Autodesk Fusion 360 part; units mm, degrees
note: some values were not read from the file. Set by a fixed rule: which sketch regions a step uses.
(part 2 of 2)
sketch "Sketch8" plane through (0, 0, 0) normal (1, 0, 0) x (0, 1, 0)
  spline S0 degree 3 poles (29.3326, 12.3675) (29.5623, 12.3811) (30.0065, 12.4074) (30.3868, 12.6373) (30.5704, 12.7484) knots 0 0 0 0 0.067871 0.131252 0.131252 0.131252 0.131252
  spline S1 degree 3 poles (30.5704, 12.7484) (30.736, 12.9046) (31.0986, 13.2469) (31.2831, 13.7117) (31.3834, 13.9642) knots 0 0 0 0 0.067501 0.147835 0.147835 0.147835 0.147835
  line L0 (31.3834, 13.9642) -> (32.7457, 13.7957)
  spline S2 degree 3 poles (32.7457, 13.7957) (32.6206, 13.424) (32.3783, 12.7048) (31.8211, 12.191) (31.5519, 11.9427) knots 0 0 0 0 0.115551 0.223613 0.223613 0.223613 0.223613
  spline S3 degree 3 poles (31.5519, 11.9427) (31.2294, 11.7506) (30.5449, 11.3428) (29.7472, 11.304) (29.3253, 11.2835) knots 0 0 0 0 0.110875 0.235384 0.235384 0.235384 0.235384
  spline S4 degree 3 poles (29.3253, 11.2835) (28.7944, 11.3187) (27.7792, 11.386) (26.9937, 12.0282) (26.619, 12.3345) knots 0 0 0 0 0.155225 0.296837 0.296837 0.296837 0.296837
  spline S5 degree 3 poles (26.619, 12.3345) (26.3278, 12.7407) (25.6988, 13.6182) (25.647, 14.701) (25.6192, 15.2825) knots 0 0 0 0 0.146839 0.31723 0.31723 0.31723 0.31723
  spline S6 degree 3 poles (25.6192, 15.2825) (25.6467, 15.8834) (25.6976, 16.9987) (26.3357, 17.9094) (26.63, 18.3294) knots 0 0 0 0 0.176138 0.326947 0.326947 0.326947 0.326947
  spline S7 degree 3 poles (26.63, 18.3294) (26.998, 18.6455) (27.752, 19.2931) (28.7442, 19.3727) (29.2521, 19.4134) knots 0 0 0 0 0.141726 0.290335 0.290335 0.290335 0.290335
  spline S8 degree 3 poles (29.2521, 19.4134) (29.7447, 19.3729) (30.7102, 19.2935) (31.4423, 18.6611) (31.8009, 18.3514) knots 0 0 0 0 0.144189 0.28257 0.28257 0.28257 0.28257
  spline S9 degree 3 poles (31.8009, 18.3514) (32.0888, 17.9395) (32.7134, 17.046) (32.763, 15.9525) (32.7897, 15.3631) knots 0 0 0 0 0.147764 0.320562 0.320562 0.320562 0.320562
  spline S10 degree 3 poles (32.7897, 15.3631) (32.7892, 15.3143) (32.7881, 15.1971) (32.7845, 15.0799) (32.7823, 15.0115) knots 0 0 0 0 0.01465 0.035165 0.035165 0.035165 0.035165
  line L1 (32.7823, 15.0115) -> (26.9816, 15.0115)
  spline S11 degree 3 poles (26.9816, 15.0115) (27.0197, 14.621) (27.0899, 13.9004) (27.5129, 13.3162) (27.7067, 13.0487) knots 0 0 0 0 0.115238 0.212619 0.212619 0.212619 0.212619
  spline S12 degree 3 poles (27.7067, 13.0487) (27.9388, 12.85) (28.4075, 12.449) (29.0224, 12.3948) (29.3326, 12.3675) knots 0 0 0 0 0.089299 0.180262 0.180262 0.180262 0.180262
  line L2 (61.3028, 12.9608) -> (61.3028, 11.4593)
  line L3 (61.3028, 11.4593) -> (59.7867, 11.4593)
  line L4 (59.7867, 11.4593) -> (59.7867, 12.9608)
  line L5 (59.7867, 12.9608) -> (61.3028, 12.9608)
  spline S13 degree 3 poles (54.2203, 11.2762) (53.7345, 11.3177) (52.7869, 11.3986) (52.1108, 12.0648) (51.7814, 12.3895) knots 0 0 0 0 0.141377 0.275753 0.275753 0.275753 0.275753
  spline S14 degree 3 poles (51.7814, 12.3895) (51.4733, 12.9652) (50.7483, 14.3203) (50.7299, 15.8658) (50.7193, 16.7547) knots 0 0 0 0 0.193319 0.455045 0.455045 0.455045 0.455045
  spline S15 degree 3 poles (50.7193, 16.7547) (50.7271, 17.3309) (50.7411, 18.3686) (50.9973, 19.3732) (51.1112, 19.8199) knots 0 0 0 0 0.172123 0.309967 0.309967 0.309967 0.309967
  spline S16 degree 3 poles (51.1112, 19.8199) (51.25, 20.1782) (51.5131, 20.8578) (52.0309, 21.369) (52.2757, 21.6107) knots 0 0 0 0 0.113767 0.215777 0.215777 0.215777 0.215777
  spline S17 degree 3 poles (52.2757, 21.6107) (52.5579, 21.7943) (53.1481, 22.1784) (53.8526, 22.2192) (54.2203, 22.2405) knots 0 0 0 0 0.099218 0.207577 0.207577 0.207577 0.207577
  spline S18 degree 3 poles (54.2203, 22.2405) (54.4947, 22.2286) (55.0219, 22.2056) (55.5048, 21.9941) (55.7364, 21.8926) knots 0 0 0 0 0.081581 0.15675 0.15675 0.15675 0.15675
  spline S19 degree 3 poles (55.7364, 21.8926) (55.9453, 21.7623) (56.3691, 21.4978) (56.6637, 21.094) (56.8131, 20.8892) knots 0 0 0 0 0.073116 0.148395 0.148395 0.148395 0.148395
  spline S20 degree 3 poles (56.8131, 20.8892) (56.949, 20.651) (57.2368, 20.1465) (57.3957, 19.5875) (57.4796, 19.2926) knots 0 0 0 0 0.081981 0.173584 0.173584 0.173584 0.173584
  spline S21 degree 3 poles (57.4796, 19.2926) (57.5498, 18.9252) (57.71, 18.0874) (57.7172, 17.234) (57.7213, 16.7547) knots 0 0 0 0 0.111981 0.255389 0.255389 0.255389 0.255389
  spline S22 degree 3 poles (57.7213, 16.7547) (57.7135, 16.1822) (57.6993, 15.1497) (57.446, 14.1497) (57.3331, 13.7042) knots 0 0 0 0 0.171021 0.308449 0.308449 0.308449 0.308449
  spline S23 degree 3 poles (57.3331, 13.7042) (57.1953, 13.3456) (56.9337, 12.665) (56.4168, 12.1523) (56.1722, 11.9097) knots 0 0 0 0 0.113733 0.215887 0.215887 0.215887 0.215887
  spline S24 degree 3 poles (56.1722, 11.9097) (55.8896, 11.7251) (55.2975, 11.3382) (54.59, 11.2975) (54.2203, 11.2762) knots 0 0 0 0 0.09951 0.208425 0.208425 0.208425 0.208425
  line L6 (61.3614, 19.8162) -> (60.9806, 14.1253)
  line L7 (60.9806, 14.1253) -> (60.131, 14.1253)
  line L8 (60.131, 14.1253) -> (59.7281, 19.8162)
  line L9 (59.7281, 19.8162) -> (59.7281, 22.1966)
  line L10 (59.7281, 22.1966) -> (61.3614, 22.1966)
  line L11 (61.3614, 22.1966) -> (61.3614, 19.8162)
  line L12 (49.5621, 12.7264) -> (49.5621, 11.4593)
  line L13 (49.5621, 11.4593) -> (42.8531, 11.4593)
  line L14 (42.8531, 11.4593) -> (42.8531, 22.1966)
  line L15 (42.8531, 22.1966) -> (44.274, 22.1966)
  line L16 (44.274, 22.1966) -> (44.274, 12.7264)
  line L17 (44.274, 12.7264) -> (49.5621, 12.7264)
  line L18 (41.2198, 12.7264) -> (41.2198, 11.4593)
  line L19 (41.2198, 11.4593) -> (34.5109, 11.4593)
  line L20 (34.5109, 11.4593) -> (34.5109, 22.1966)
  line L21 (34.5109, 22.1966) -> (35.9317, 22.1966)
  line L22 (35.9317, 22.1966) -> (35.9317, 12.7264)
  line L23 (35.9317, 12.7264) -> (41.2198, 12.7264)
  line L24 (16.8595, 16.5203) -> (16.8595, 11.4593)
  line L25 (16.8595, 11.4593) -> (15.4386, 11.4593)
  line L26 (15.4386, 11.4593) -> (15.4386, 22.1966)
  line L27 (15.4386, 22.1966) -> (16.8595, 22.1966)
  line L28 (16.8595, 22.1966) -> (16.8595, 17.7874)
  line L29 (16.8595, 17.7874) -> (22.4405, 17.7874)
  line L30 (22.4405, 17.7874) -> (22.4405, 22.1966)
  line L31 (22.4405, 22.1966) -> (23.8614, 22.1966)
  line L32 (23.8614, 22.1966) -> (23.8614, 11.4593)
  line L33 (23.8614, 11.4593) -> (22.4405, 11.4593)
  line L34 (22.4405, 11.4593) -> (22.4405, 16.5203)
  line L35 (22.4405, 16.5203) -> (16.8595, 16.5203)
  line L36 (24.5, 46.5) -> (51.5, 46.5)
  line L37 (51.5, 46.5) -> (51.5, 43.5)
  arc A0 (44.0625, 39.115) -> (51.5, 43.5) centre (51.5, 35) ccw
  line L38 (44.0625, 39.115) -> (31.9375, 39.115)
  arc A1 (24.5, 43.5) -> (31.9375, 39.115) centre (24.5, 35) ccw
  line L39 (24.5, 43.5) -> (24.5, 46.5)
  line L40 (63, 56) -> (53, 56)
  line L41 (53, 56) -> (53, 53)
  line L42 (53, 53) -> (43, 53)
  line L43 (43, 53) -> (43, 56)
  line L44 (43, 56) -> (33, 56)
  line L45 (33, 56) -> (33, 53)
  line L46 (33, 53) -> (23, 53)
  line L47 (23, 53) -> (23, 56)
  line L48 (23, 56) -> (13, 56)
  line L49 (13, 56) -> (13, 53)
  line L50 (13, 53) -> (3, 53)
  line L51 (3, 53) -> (3, 56)
  line L52 (3, 56) -> (0, 56)
  line L53 (0, 56) -> (0, 43)
  line L54 (0, 43) -> (3, 43)
  line L55 (3, 43) -> (3, 33)
  line L56 (3, 33) -> (0, 33)
  line L57 (0, 33) -> (0, 23)
  line L58 (0, 23) -> (3, 23)
  line L59 (3, 23) -> (3, 13)
  line L60 (3, 13) -> (0, 13)
  line L61 (0, 13) -> (0, 0)
  line L62 (0, 0) -> (3, 0)
  line L63 (3, 0) -> (3, 3)
  line L64 (3, 3) -> (13, 3)
  line L65 (13, 3) -> (13, 0)
  line L66 (13, 0) -> (23, 0)
  line L67 (23, 0) -> (23, 3)
  line L68 (23, 3) -> (33, 3)
  line L69 (33, 3) -> (33, 0)
  line L70 (33, 0) -> (43, 0)
  line L71 (43, 0) -> (43, 3)
  line L72 (43, 3) -> (53, 3)
  line L73 (53, 3) -> (53, 0)
  line L74 (53, 0) -> (63, 0)
  line L75 (63, 0) -> (63, 3)
  line L76 (63, 3) -> (73, 3)
  line L77 (73, 3) -> (73, 0)
  line L78 (73, 0) -> (76, 0)
  line L79 (76, 0) -> (76, 13)
  line L80 (76, 13) -> (73, 13)
  line L81 (73, 13) -> (73, 23)
  line L82 (73, 23) -> (76, 23)
  line L83 (76, 23) -> (76, 33)
  line L84 (76, 33) -> (73, 33)
  line L85 (73, 33) -> (73, 43)
  line L86 (73, 43) -> (76, 43)
  line L87 (76, 43) -> (76, 56)
  line L88 (76, 56) -> (73, 56)
  line L89 (73, 56) -> (73, 53)
  line L90 (73, 53) -> (63, 53)
  line L91 (63, 53) -> (63, 56)
sketch "Sketch9" plane through (0, 76, 0) normal (0, 1, 0) x (-1, 0, 0)
  line L0 (183, 0) -> (193, 0)
  line L1 (193, 0) -> (193, 13)
  line L2 (193, 13) -> (196, 13)
  line L3 (196, 13) -> (196, 23)
  line L4 (196, 23) -> (193, 23)
  line L5 (193, 23) -> (193, 33)
  line L6 (193, 33) -> (196, 33)
  line L7 (196, 33) -> (196, 43)
  line L8 (196, 43) -> (193, 43)
  line L9 (193, 43) -> (193, 56)
  line L10 (193, 56) -> (183, 56)
  line L11 (183, 56) -> (183, 53)
  line L12 (183, 53) -> (173, 53)
  line L13 (173, 53) -> (173, 56)
  line L14 (173, 56) -> (163, 56)
  line L15 (163, 56) -> (163, 53)
  line L16 (163, 53) -> (153, 53)
  line L17 (153, 53) -> (153, 56)
  line L18 (153, 56) -> (143, 56)
  line L19 (143, 56) -> (143, 53)
  line L20 (143, 53) -> (133, 53)
  line L21 (133, 53) -> (133, 56)
  line L22 (133, 56) -> (123, 56)
  line L23 (123, 56) -> (123, 53)
  line L24 (123, 53) -> (113, 53)
  line L25 (113, 53) -> (113, 56)
  line L26 (113, 56) -> (103, 56)
  line L27 (103, 56) -> (103, 53)
  line L28 (103, 53) -> (93, 53)
  line L29 (93, 53) -> (93, 56)
  line L30 (93, 56) -> (83, 56)
  line L31 (83, 56) -> (83, 53)
  line L32 (83, 53) -> (73, 53)
  line L33 (73, 53) -> (73, 56)
  line L34 (73, 56) -> (63, 56)
  line L35 (63, 56) -> (63, 53)
  line L36 (63, 53) -> (53, 53)
  line L37 (53, 53) -> (53, 56)
  line L38 (53, 56) -> (43, 56)
  line L39 (43, 56) -> (43, 53)
  line L40 (43, 53) -> (33, 53)
  line L41 (33, 53) -> (33, 56)
  line L42 (33, 56) -> (23, 56)
  line L43 (23, 56) -> (23, 53)
  line L44 (23, 53) -> (13, 53)
  line L45 (13, 53) -> (13, 56)
  line L46 (13, 56) -> (3, 56)
  line L47 (3, 56) -> (3, 43)
  line L48 (3, 43) -> (0, 43)
  line L49 (0, 43) -> (0, 33)
  line L50 (0, 33) -> (3, 33)
  line L51 (3, 33) -> (3, 23)
  line L52 (3, 23) -> (0, 23)
  line L53 (0, 23) -> (0, 13)
  line L54 (0, 13) -> (3, 13)
  line L55 (3, 13) -> (3, 0)
  line L56 (3, 0) -> (13, 0)
  line L57 (13, 0) -> (13, 3)
  line L58 (13, 3) -> (23, 3)
  line L59 (23, 3) -> (23, 0)
  line L60 (23, 0) -> (33, 0)
  line L61 (33, 0) -> (33, 3)
  line L62 (33, 3) -> (43, 3)
  line L63 (43, 3) -> (43, 0)
  line L64 (43, 0) -> (53, 0)
  line L65 (53, 0) -> (53, 3)
  line L66 (53, 3) -> (63, 3)
  line L67 (63, 3) -> (63, 0)
  line L68 (63, 0) -> (73, 0)
  line L69 (73, 0) -> (73, 3)
  line L70 (73, 3) -> (83, 3)
  line L71 (83, 3) -> (83, 0)
  line L72 (83, 0) -> (93, 0)
  line L73 (93, 0) -> (93, 3)
  line L74 (93, 3) -> (103, 3)
  line L75 (103, 3) -> (103, 0)
  line L76 (103, 0) -> (113, 0)
  line L77 (113, 0) -> (113, 3)
  line L78 (113, 3) -> (123, 3)
  line L79 (123, 3) -> (123, 0)
  line L80 (123, 0) -> (133, 0)
  line L81 (133, 0) -> (133, 3)
  line L82 (133, 3) -> (143, 3)
  line L83 (143, 3) -> (143, 0)
  line L84 (143, 0) -> (153, 0)
  line L85 (153, 0) -> (153, 3)
  line L86 (153, 3) -> (163, 3)
  line L87 (163, 3) -> (163, 0)
  line L88 (163, 0) -> (173, 0)
  line L89 (173, 0) -> (173, 3)
  line L90 (173, 3) -> (183, 3)
  line L91 (183, 3) -> (183, 0)
  line L92 (95, 15) -> (10, 15)
  line L93 (10, 15) -> (10, 18)
  line L94 (10, 18) -> (95, 18)
  line L95 (95, 18) -> (95, 15)
  line L96 (186, 33) -> (115, 33)
  line L97 (115, 33) -> (115, 36)
  line L98 (115, 36) -> (186, 36)
  line L99 (186, 36) -> (186, 33)
  line L100 (187, 50) -> (187, 49)
  line L101 (187, 49) -> (180, 49)
  line L102 (180, 49) -> (180, 50)
  line L103 (180, 50) -> (187, 50)
sketch "Sketch11" plane through (0, 0, 56) normal (0, 0, 1) x (-1, 0, 0)
  line L0 (32, -68) -> (32, -48)
  line L1 (32, -48) -> (90, -48)
  line L2 (90, -48) -> (90, -68)
  line L3 (90, -68) -> (32, -68)
  line L4 (7.3818, -6.8746) -> (8.8818, -6.8746)
  line L5 (8.8818, -6.8746) -> (8.8818, -12.8746)
  line L6 (8.8818, -12.8746) -> (7.3818, -12.8746)
  line L7 (7.3818, -12.8746) -> (7.3818, -6.8746)
  line L8 (13, -3) -> (0, -3)
  line L9 (0, -3) -> (0, -13)
  line L10 (0, -13) -> (3, -13)
  line L11 (3, -13) -> (3, -23)
  line L12 (3, -23) -> (0, -23)
  line L13 (0, -23) -> (0, -33)
  line L14 (0, -33) -> (3, -33)
  line L15 (3, -33) -> (3, -43)
  line L16 (3, -43) -> (0, -43)
  line L17 (0, -43) -> (0, -53)
  line L18 (0, -53) -> (3, -53)
  line L19 (3, -53) -> (3, -63)
  line L20 (3, -63) -> (0, -63)
  line L21 (0, -63) -> (0, -73)
  line L22 (0, -73) -> (13, -73)
  line L23 (13, -73) -> (13, -76)
  line L24 (13, -76) -> (23, -76)
  line L25 (23, -76) -> (23, -73)
  line L26 (23, -73) -> (33, -73)
  line L27 (33, -73) -> (33, -76)
  line L28 (33, -76) -> (43, -76)
  line L29 (43, -76) -> (43, -73)
  line L30 (43, -73) -> (53, -73)
  line L31 (53, -73) -> (53, -76)
  line L32 (53, -76) -> (63, -76)
  line L33 (63, -76) -> (63, -73)
  line L34 (63, -73) -> (73, -73)
  line L35 (73, -73) -> (73, -76)
  line L36 (73, -76) -> (83, -76)
  line L37 (83, -76) -> (83, -73)
  line L38 (83, -73) -> (93, -73)
  line L39 (93, -73) -> (93, -76)
  line L40 (93, -76) -> (103, -76)
  line L41 (103, -76) -> (103, -73)
  line L42 (103, -73) -> (113, -73)
  line L43 (113, -73) -> (113, -76)
  line L44 (113, -76) -> (123, -76)
  line L45 (123, -76) -> (123, -73)
  line L46 (123, -73) -> (133, -73)
  line L47 (133, -73) -> (133, -76)
  line L48 (133, -76) -> (143, -76)
  line L49 (143, -76) -> (143, -73)
  line L50 (143, -73) -> (153, -73)
  line L51 (153, -73) -> (153, -76)
  line L52 (153, -76) -> (163, -76)
  line L53 (163, -76) -> (163, -73)
  line L54 (163, -73) -> (173, -73)
  line L55 (173, -73) -> (173, -76)
  line L56 (173, -76) -> (183, -76)
  line L57 (183, -76) -> (183, -73)
  line L58 (183, -73) -> (196, -73)
  line L59 (196, -73) -> (196, -63)
  line L60 (196, -63) -> (193, -63)
  line L61 (193, -63) -> (193, -53)
  line L62 (193, -53) -> (196, -53)
  line L63 (196, -53) -> (196, -43)
  line L64 (196, -43) -> (193, -43)
  line L65 (193, -43) -> (193, -33)
  line L66 (193, -33) -> (196, -33)
  line L67 (196, -33) -> (196, -23)
  line L68 (196, -23) -> (193, -23)
  line L69 (193, -23) -> (193, -13)
  line L70 (193, -13) -> (196, -13)
  line L71 (196, -13) -> (196, -3)
  line L72 (196, -3) -> (183, -3)
  line L73 (183, -3) -> (183, 0)
  line L74 (183, 0) -> (173, 0)
  line L75 (173, 0) -> (173, -3)
  line L76 (173, -3) -> (163, -3)
  line L77 (163, -3) -> (163, 0)
  line L78 (163, 0) -> (153, 0)
  line L79 (153, 0) -> (153, -3)
  line L80 (153, -3) -> (143, -3)
  line L81 (143, -3) -> (143, 0)
  line L82 (143, 0) -> (133, 0)
  line L83 (133, 0) -> (133, -3)
  line L84 (133, -3) -> (123, -3)
  line L85 (123, -3) -> (123, 0)
  line L86 (123, 0) -> (113, 0)
  line L87 (113, 0) -> (113, -3)
  line L88 (113, -3) -> (103, -3)
  line L89 (103, -3) -> (103, 0)
  line L90 (103, 0) -> (93, 0)
  line L91 (93, 0) -> (93, -3)
  line L92 (93, -3) -> (83, -3)
  line L93 (83, -3) -> (83, 0)
  line L94 (83, 0) -> (73, 0)
  line L95 (73, 0) -> (73, -3)
  line L96 (73, -3) -> (63, -3)
  line L97 (63, -3) -> (63, 0)
  line L98 (63, 0) -> (53, 0)
  line L99 (53, 0) -> (53, -3)
  line L100 (53, -3) -> (43, -3)
  line L101 (43, -3) -> (43, 0)
  line L102 (43, 0) -> (33, 0)
  line L103 (33, 0) -> (33, -3)
  line L104 (33, -3) -> (23, -3)
  line L105 (23, -3) -> (23, 0)
  line L106 (23, 0) -> (13, 0)
  line L107 (13, 0) -> (13, -3)
sketch "Sketch12" plane through (-196, 0, 0) normal (-1, 0, 0) x (0, -1, 0)
  line L0 (-53, 56) -> (-63, 56)
  line L1 (-63, 56) -> (-63, 53)
  line L2 (-63, 53) -> (-73, 53)
  line L3 (-73, 53) -> (-73, 56)
  line L4 (-73, 56) -> (-76, 56)
  line L5 (-76, 56) -> (-76, 43)
  line L6 (-76, 43) -> (-73, 43)
  line L7 (-73, 43) -> (-73, 33)
  line L8 (-73, 33) -> (-76, 33)
  line L9 (-76, 33) -> (-76, 23)
  line L10 (-76, 23) -> (-73, 23)
  line L11 (-73, 23) -> (-73, 13)
  line L12 (-73, 13) -> (-76, 13)
  line L13 (-76, 13) -> (-76, 0)
  line L14 (-76, 0) -> (-73, 0)
  line L15 (-73, 0) -> (-73, 3)
  line L16 (-73, 3) -> (-63, 3)
  line L17 (-63, 3) -> (-63, 0)
  line L18 (-63, 0) -> (-53, 0)
  line L19 (-53, 0) -> (-53, 3)
  line L20 (-53, 3) -> (-43, 3)
  line L21 (-43, 3) -> (-43, 0)
  line L22 (-43, 0) -> (-33, 0)
  line L23 (-33, 0) -> (-33, 3)
  line L24 (-33, 3) -> (-23, 3)
  line L25 (-23, 3) -> (-23, 0)
  line L26 (-23, 0) -> (-13, 0)
  line L27 (-13, 0) -> (-13, 3)
  line L28 (-13, 3) -> (-3, 3)
  line L29 (-3, 3) -> (-3, 0)
  line L30 (-3, 0) -> (0, 0)
  line L31 (0, 0) -> (0, 13)
  line L32 (0, 13) -> (-3, 13)
  line L33 (-3, 13) -> (-3, 23)
  line L34 (-3, 23) -> (0, 23)
  line L35 (0, 23) -> (0, 33)
  line L36 (0, 33) -> (-3, 33)
  line L37 (-3, 33) -> (-3, 43)
  line L38 (-3, 43) -> (0, 43)
  line L39 (0, 43) -> (0, 56)
  line L40 (0, 56) -> (-3, 56)
  line L41 (-3, 56) -> (-3, 53)
  line L42 (-3, 53) -> (-13, 53)
  line L43 (-13, 53) -> (-13, 56)
  line L44 (-13, 56) -> (-23, 56)
  line L45 (-23, 56) -> (-23, 53)
  line L46 (-23, 53) -> (-33, 53)
  line L47 (-33, 53) -> (-33, 56)
  line L48 (-33, 56) -> (-43, 56)
  line L49 (-43, 56) -> (-43, 53)
  line L50 (-43, 53) -> (-53, 53)
  line L51 (-53, 53) -> (-53, 56)
sketch "Sketch13" plane through (0, 0, 0) normal (0, 0, -1) x (1, 0, 0)
  line L0 (0, -3) -> (-13, -3)
  line L1 (-13, -3) -> (-13, 0)
  line L2 (-13, 0) -> (-23, 0)
  line L3 (-23, 0) -> (-23, -3)
  line L4 (-23, -3) -> (-33, -3)
  line L5 (-33, -3) -> (-33, 0)
  line L6 (-33, 0) -> (-43, 0)
  line L7 (-43, 0) -> (-43, -3)
  line L8 (-43, -3) -> (-53, -3)
  line L9 (-53, -3) -> (-53, 0)
  line L10 (-53, 0) -> (-63, 0)
  line L11 (-63, 0) -> (-63, -3)
  line L12 (-63, -3) -> (-73, -3)
  line L13 (-73, -3) -> (-73, 0)
  line L14 (-73, 0) -> (-83, 0)
  line L15 (-83, 0) -> (-83, -3)
  line L16 (-83, -3) -> (-93, -3)
  line L17 (-93, -3) -> (-93, 0)
  line L18 (-93, 0) -> (-103, 0)
  line L19 (-103, 0) -> (-103, -3)
  line L20 (-103, -3) -> (-113, -3)
  line L21 (-113, -3) -> (-113, 0)
  line L22 (-113, 0) -> (-123, 0)
  line L23 (-123, 0) -> (-123, -3)
  line L24 (-123, -3) -> (-133, -3)
  line L25 (-133, -3) -> (-133, 0)
  line L26 (-133, 0) -> (-143, 0)
  line L27 (-143, 0) -> (-143, -3)
  line L28 (-143, -3) -> (-153, -3)
  line L29 (-153, -3) -> (-153, 0)
  line L30 (-153, 0) -> (-163, 0)
  line L31 (-163, 0) -> (-163, -3)
  line L32 (-163, -3) -> (-173, -3)
  line L33 (-173, -3) -> (-173, 0)
  line L34 (-173, 0) -> (-183, 0)
  line L35 (-183, 0) -> (-183, -3)
  line L36 (-183, -3) -> (-196, -3)
  line L37 (-196, -3) -> (-196, -13)
  line L38 (-196, -13) -> (-193, -13)
  line L39 (-193, -13) -> (-193, -23)
  line L40 (-193, -23) -> (-196, -23)
  line L41 (-196, -23) -> (-196, -33)
  line L42 (-196, -33) -> (-193, -33)
  line L43 (-193, -33) -> (-193, -43)
  line L44 (-193, -43) -> (-196, -43)
  line L45 (-196, -43) -> (-196, -53)
  line L46 (-196, -53) -> (-193, -53)
  line L47 (-193, -53) -> (-193, -63)
  line L48 (-193, -63) -> (-196, -63)
  line L49 (-196, -63) -> (-196, -73)
  line L50 (-196, -73) -> (-183, -73)
  line L51 (-183, -73) -> (-183, -76)
  line L52 (-183, -76) -> (-173, -76)
  line L53 (-173, -76) -> (-173, -73)
  line L54 (-173, -73) -> (-163, -73)
  line L55 (-163, -73) -> (-163, -76)
  line L56 (-163, -76) -> (-153, -76)
  line L57 (-153, -76) -> (-153, -73)
  line L58 (-153, -73) -> (-143, -73)
  line L59 (-143, -73) -> (-143, -76)
  line L60 (-143, -76) -> (-133, -76)
  line L61 (-133, -76) -> (-133, -73)
  line L62 (-133, -73) -> (-123, -73)
  line L63 (-123, -73) -> (-123, -76)
  line L64 (-123, -76) -> (-113, -76)
  line L65 (-113, -76) -> (-113, -73)
  line L66 (-113, -73) -> (-103, -73)
  line L67 (-103, -73) -> (-103, -76)
  line L68 (-103, -76) -> (-93, -76)
  line L69 (-93, -76) -> (-93, -73)
  line L70 (-93, -73) -> (-83, -73)
  line L71 (-83, -73) -> (-83, -76)
  line L72 (-83, -76) -> (-73, -76)
  line L73 (-73, -76) -> (-73, -73)
  line L74 (-73, -73) -> (-63, -73)
  line L75 (-63, -73) -> (-63, -76)
  line L76 (-63, -76) -> (-53, -76)
  line L77 (-53, -76) -> (-53, -73)
  line L78 (-53, -73) -> (-43, -73)
  line L79 (-43, -73) -> (-43, -76)
  line L80 (-43, -76) -> (-33, -76)
  line L81 (-33, -76) -> (-33, -73)
  line L82 (-33, -73) -> (-23, -73)
  line L83 (-23, -73) -> (-23, -76)
  line L84 (-23, -76) -> (-13, -76)
  line L85 (-13, -76) -> (-13, -73)
  line L86 (-13, -73) -> (0, -73)
  line L87 (0, -73) -> (0, -63)
  line L88 (0, -63) -> (-3, -63)
  line L89 (-3, -63) -> (-3, -53)
  line L90 (-3, -53) -> (0, -53)
  line L91 (0, -53) -> (0, -43)
  line L92 (0, -43) -> (-3, -43)
  line L93 (-3, -43) -> (-3, -33)
  line L94 (-3, -33) -> (0, -33)
  line L95 (0, -33) -> (0, -23)
  line L96 (0, -23) -> (-3, -23)
  line L97 (-3, -23) -> (-3, -13)
  line L98 (-3, -13) -> (0, -13)
  line L99 (0, -13) -> (0, -3)
sketch "Sketch14" plane through (0, 76, 0) normal (0, 1, 0) x (-1, 0, 0)
  line L0 (95, 15) -> (10, 15)
  line L1 (10, 15) -> (10, 18)
  line L2 (10, 18) -> (95, 18)
  line L3 (95, 18) -> (95, 15)
  line L4 (186, 33) -> (115, 33)
  line L5 (115, 33) -> (115, 36)
  line L6 (115, 36) -> (186, 36)
  line L7 (186, 36) -> (186, 33)
  line L8 (187, 50) -> (187, 49)
  line L9 (187, 49) -> (180, 49)
  line L10 (180, 49) -> (180, 50)
  line L11 (180, 50) -> (187, 50)
  line L12 (183, 0) -> (193, 0)
  line L13 (193, 0) -> (193, 13)
  line L14 (193, 13) -> (196, 13)
  line L15 (196, 13) -> (196, 23)
  line L16 (196, 23) -> (193, 23)
  line L17 (193, 23) -> (193, 33)
  line L18 (193, 33) -> (196, 33)
  line L19 (196, 33) -> (196, 43)
  line L20 (196, 43) -> (193, 43)
  line L21 (193, 43) -> (193, 56)
  line L22 (193, 56) -> (183, 56)
  line L23 (183, 56) -> (183, 53)
  line L24 (183, 53) -> (173, 53)
  line L25 (173, 53) -> (173, 56)
  line L26 (173, 56) -> (163, 56)
  line L27 (163, 56) -> (163, 53)
  line L28 (163, 53) -> (153, 53)
  line L29 (153, 53) -> (153, 56)
  line L30 (153, 56) -> (143, 56)
  line L31 (143, 56) -> (143, 53)
  line L32 (143, 53) -> (133, 53)
  line L33 (133, 53) -> (133, 56)
  line L34 (133, 56) -> (123, 56)
  line L35 (123, 56) -> (123, 53)
  line L36 (123, 53) -> (113, 53)
  line L37 (113, 53) -> (113, 56)
  line L38 (113, 56) -> (103, 56)
  line L39 (103, 56) -> (103, 53)
  line L40 (103, 53) -> (93, 53)
  line L41 (93, 53) -> (93, 56)
  line L42 (93, 56) -> (83, 56)
  line L43 (83, 56) -> (83, 53)
  line L44 (83, 53) -> (73, 53)
  line L45 (73, 53) -> (73, 56)
  line L46 (73, 56) -> (63, 56)
  line L47 (63, 56) -> (63, 53)
  line L48 (63, 53) -> (53, 53)
  line L49 (53, 53) -> (53, 56)
  line L50 (53, 56) -> (43, 56)
  line L51 (43, 56) -> (43, 53)
  line L52 (43, 53) -> (33, 53)
  line L53 (33, 53) -> (33, 56)
  line L54 (33, 56) -> (23, 56)
  line L55 (23, 56) -> (23, 53)
  line L56 (23, 53) -> (13, 53)
  line L57 (13, 53) -> (13, 56)
  line L58 (13, 56) -> (3, 56)
  line L59 (3, 56) -> (3, 43)
  line L60 (3, 43) -> (0, 43)
  line L61 (0, 43) -> (0, 33)
  line L62 (0, 33) -> (3, 33)
  line L63 (3, 33) -> (3, 23)
  line L64 (3, 23) -> (0, 23)
  line L65 (0, 23) -> (0, 13)
  line L66 (0, 13) -> (3, 13)
  line L67 (3, 13) -> (3, 0)
  line L68 (3, 0) -> (13, 0)
  line L69 (13, 0) -> (13, 3)
  line L70 (13, 3) -> (23, 3)
  line L71 (23, 3) -> (23, 0)
  line L72 (23, 0) -> (33, 0)
  line L73 (33, 0) -> (33, 3)
  line L74 (33, 3) -> (43, 3)
  line L75 (43, 3) -> (43, 0)
  line L76 (43, 0) -> (53, 0)
  line L77 (53, 0) -> (53, 3)
  line L78 (53, 3) -> (63, 3)
  line L79 (63, 3) -> (63, 0)
  line L80 (63, 0) -> (73, 0)
  line L81 (73, 0) -> (73, 3)
  line L82 (73, 3) -> (83, 3)
  line L83 (83, 3) -> (83, 0)
  line L84 (83, 0) -> (93, 0)
  line L85 (93, 0) -> (93, 3)
  line L86 (93, 3) -> (103, 3)
  line L87 (103, 3) -> (103, 0)
  line L88 (103, 0) -> (113, 0)
  line L89 (113, 0) -> (113, 3)
  line L90 (113, 3) -> (123, 3)
  line L91 (123, 3) -> (123, 0)
  line L92 (123, 0) -> (133, 0)
  line L93 (133, 0) -> (133, 3)
  line L94 (133, 3) -> (143, 3)
  line L95 (143, 3) -> (143, 0)
  line L96 (143, 0) -> (153, 0)
  line L97 (153, 0) -> (153, 3)
  line L98 (153, 3) -> (163, 3)
  line L99 (163, 3) -> (163, 0)
  line L100 (163, 0) -> (173, 0)
  line L101 (173, 0) -> (173, 3)
  line L102 (173, 3) -> (183, 3)
  line L103 (183, 3) -> (183, 0)
equation "Fingerlength = 10 mm"
equation "Fingerheight = 3 mm"
equation "height = 56 mm"
equation "width = 76 mm"
equation "length = 196 mm"
equation "thickness = 3 mm"
equation "d7 = length"
equation "d8 = width"
equation "d9 = thickness"
equation "d11 = width"
equation "d12 = height"
equation "d13 = thickness"
equation "d14 = thickness"
equation "d15 = Fingerheight"
equation "d16 = Fingerlength"
equation "d17 = Fingerheight"
equation "d18 = Fingerlength"
equation "d19 = Fingerheight"
equation "d20 = Fingerlength"
equation "d21 = Fingerheight"
equation "d22 = Fingerlength"
equation "d23 = Fingerheight"
equation "d24 = Fingerlength"
equation "d47 = width / 2"
equation "d48 = height"
equation "d49 = thickness"
equation "d50 = thickness"
equation "d51 = Fingerlength"
equation "d52 = Fingerheight"
equation "d53 = Fingerlength"
equation "d54 = Fingerheight"
equation "d55 = Fingerlength"
equation "d56 = Fingerheight"
equation "d57 = Fingerlength"
equation "d58 = Fingerheight"
equation "d59 = Fingerlength"
equation "d60 = Fingerheight"
equation "d61 = Fingerlength"
equation "d62 = Fingerheight"
equation "d63 = Fingerlength"
equation "d64 = Fingerheight"
equation "d65 = thickness"
equation "d66 = thickness"
equation "d67 = -thickness"
equation "d69 = length"
equation "d70 = height"
equation "d71 = thickness"
equation "d72 = thickness"
equation "d73 = Fingerheight"
equation "d74 = Fingerlength"
equation "d75 = Fingerheight"
equation "d76 = Fingerlength"
equation "d77 = thickness"
equation "d78 = thickness"
equation "d79 = Fingerheight"
equation "d80 = Fingerlength"
equation "d81 = Fingerheight"
equation "d82 = Fingerlength"
equation "d83 = Fingerlength"
equation "d84 = Fingerheight"
equation "d85 = Fingerlength"
equation "d86 = Fingerheight"
equation "d87 = Fingerlength"
equation "d88 = Fingerheight"
equation "d89 = Fingerlength"
equation "d90 = Fingerheight"
equation "d91 = Fingerlength"
equation "d92 = Fingerheight"
equation "d93 = Fingerlength"
equation "d94 = Fingerheight"
equation "d95 = Fingerlength"
equation "d96 = Fingerheight"
equation "d97 = Fingerlength"
equation "d98 = Fingerheight"
equation "d99 = Fingerlength"
equation "d100 = Fingerheight"
equation "d101 = Fingerlength"
equation "d102 = Fingerheight"
equation "d103 = Fingerlength"
equation "d104 = Fingerlength"
equation "d105 = Fingerheight"
equation "d106 = Fingerlength"
equation "d107 = Fingerheight"
equation "d108 = Fingerlength"
equation "d109 = Fingerheight"
equation "d110 = Fingerlength"
equation "d111 = Fingerheight"
equation "d112 = Fingerlength"
equation "d113 = Fingerheight"
equation "d114 = Fingerlength"
equation "d115 = Fingerheight"
equation "d116 = Fingerlength"
equation "d117 = Fingerheight"
equation "d118 = Fingerlength"
equation "d119 = Fingerheight"
equation "d120 = thickness"
equation "d121 = thickness"
equation "d122 = ( 196 / 2 ) * 1 mm"
equation "d123 = Fingerheight"
equation "d124 = Fingerlength"
equation "d125 = -thickness"
equation "d127 = -length / 2"
equation "d129 = -width / 2"
equation "d131 = -height / 2"
equation "d133 = width / 2"
equation "d141 = -thickness"
equation "d151 = -thickness"
equation "d158 = -thickness"
equation "d160 = -width"
